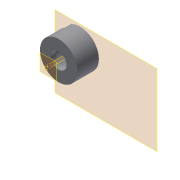
# Autodesk Inventor part: 101_Huawei_FilterLens_Adapter_Thread
Saved by Autodesk Inventor 2019 (Build 230136000, 136)
## iProperties
Created: 2019-06-17
Part Number: 101_Huawei_FilterLens_Adapter_Thread
Material: Generic
Document SubType Name: Modeling
Designer: diederichbenedict
Density: 1 g/cm^3
Appearance: Default
Author: diederichbenedict
Autodesk Inventor part; units mm, degrees
ref_plane "XZ Plane" through (0, 0, 0) normal (0, 1, 0) x (-1, 0, 0)
ref_plane "XY Plane" through (0, 0, 0) normal (0, 0, 1) x (1, 0, 0)
ref_plane "Work Plane1" through (0, 0, 0) normal (0, 0, 1) x (1, 0, 0)
ref_plane "Work Plane2" through (0, -6, 25.4) normal (0, 0, 1) x (1, 0, 0)
sketch "Sketch1" plane through (0, -6, 25.4) normal (0, 0, 1) x (1, 0, 0)
  point P0 (0, 6)
  point P1 (0, 6)
  constraints: 1 coincident
ref_plane "Work Plane3" through (0, 0, 25.4) normal (1, 0, 0) x (0, 1, 0)
sketch "Sketch2" plane through (0, 0, 25.4) normal (1, 0, 0) x (0, 1, 0)
  line L0 (12.6, -22.1) -> (12.6, -27.1) construction
  line L1 (8.75, -15.4) -> (8.75, -20.1) construction
  line L2 (-8.75, -15.4) -> (8.75, -15.4) construction
  arc A0 (-8.75, -20.1) -> (8.75, -20.1) centre (0, 0) ccw construction
  line L3 (-6, 0) -> (6, 0) construction
  line L4 (12.8, -25.4) -> (12.8, -21.9)
  line L5 (9.75, -20.7) -> (9.75, -15.0193)
  line L6 (9.75, -15.0193) -> (9.75, -12.4)
  line L7 (9.75, -12.4) -> (6.2, -12.4)
  line L8 (6.2, -12.4) -> (6.2, -8.4)
  line L9 (6.2, -8.4) -> (14.8, -8.4)
  line L10 (14.8, -8.4) -> (14.8, -25.4)
  line L11 (14.8, -25.4) -> (12.8, -25.4)
  line L12 (6, 0) -> (6, -15.4)
  line L13 (0, 0) -> (0, -25.4)
  line L14 (12.8, -21.9) -> (12.8, -20.7)
  line L15 (12.8, -20.7) -> (9.75, -20.7)
  line L16 (13.9634, -25.4) -> (8.8415, -25.4) projected
  dimension "d0" = 1
  dimension "d1" = 0.2
  dimension "d3" = 2
  dimension "d6" = 3
  dimension "d7" = 0.2
  dimension "d8" = 4
  dimension "d12" = 4.7
  constraints: 28 end point, 6 perpendicular, 6 vertical, 2 point on circle, 2 point on line, 1 centre point, 8 other
  measures "d0" distance between parallel lines of L1 L5
  measures "d1" distance between parallel lines of L0 L4
  measures "d3" distance between parallel lines of L4 L10
  measures "d6" distance between parallel lines of L2 L7
  measures "d7" distance between parallel lines of L12 L8
  measures "d8" distance between parallel lines of L7 L9
  measures "d12" distance between parallel lines of L15 L11
revolve "Revolution1" add sketch "Sketch2" angle 360 about axis through (0, 0, 25.4) along (0, -0.0000003, -1)
sketch "Sketch4" plane through (0, 0, 0) normal (1, 0, 0) x (0, 1, 0)
  line L0 (12.6, 3.3) -> (-12.6, 3.3) projected
  line L1 (-12.8, 0) -> (12.8, 0) projected
  line L2 (12.8, 3.3) -> (-12.8, 3.3)
  line L3 (-12.8, 3.3) -> (-12.8, 0)
  line L4 (-12.8, 0) -> (12.8, 0)
  line L5 (12.8, 0) -> (12.8, 3.3)
  line L6 (-12.8, 4.7) -> (12.8, 4.7) projected
  line L7 (-12.8, 3.3) -> (12.8, 3.3)
  line L8 (12.8, 3.3) -> (12.8, 4.7)
  line L9 (12.8, 4.7) -> (-12.8, 4.7)
  line L10 (-12.8, 4.7) -> (-12.8, 3.3)
  point P0 (0, 0)
  constraints: 16 end point, 4 parallel, 2 horizontal, 2 perpendicular
extrude "Extrusion1" cut sketch "Sketch4" against normal through all
body "Solid1"
